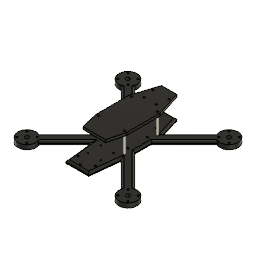
Drone Frame (Autodesk Fusion 360 design; units mm, degrees)
Autodesk Fusion 360 part; units mm, degrees
note: some values were not read from the file. Chosen so that the rebuilt part matches the saved one: which bodies a step acts on; which face or edge a step refers to; which pieces of a blend or face edit are solid. Set by a fixed rule: which sketch regions a step uses.
sketch "Sketch1" plane through (0, 0, 0) normal (0, 0, 1) x (1, 0, 0)
  line L0 (-15.25, 15.25) -> (15.25, 15.25)
  line L1 (15.25, 15.25) -> (15.25, -15.25)
  line L2 (15.25, -15.25) -> (-15.25, -15.25)
  line L3 (-15.25, -15.25) -> (-15.25, 15.25)
  circle A0 centre (-15.25, 15.25) radius 1.5
  circle A1 centre (15.25, 15.25) radius 1.5
  circle A2 centre (-15.25, -15.25) radius 1.5
  circle A3 centre (15.25, -15.25) radius 1.5
  line L4 (-23, 22) -> (0, 22)
  line L5 (-23, 22) -> (23, 22)
  line L6 (23, 22) -> (23, -22)
  line L7 (23, -22) -> (-23, -22)
  line L8 (-23, -22) -> (-23, 22)
  line L9 (-10, -38) -> (-10, -33)
  line L10 (-10, -33) -> (0, -33)
  line L11 (-10, -33) -> (10, -33)
  line L12 (10, -33) -> (10, -53)
  line L13 (10, -53) -> (-10, -53)
  line L14 (-10, -53) -> (-10, -33)
  circle A4 centre (-10, -33) radius 1
  circle A5 centre (10, -33) radius 1
  circle A6 centre (-10, -53) radius 1
  circle A7 centre (10, -53) radius 1
  line L15 (9.6, 35) -> (-9.6, 35)
  circle A8 centre (-9.6, 35) radius 1.5
  circle A9 centre (9.6, 35) radius 1.5
  circle A10 centre (0, 0) radius 112.5
  line L16 (0, 0) -> (-79.5495, -79.5495)
  line L17 (0, 0) -> (-79.5495, 79.5495)
  line L18 (0, 0) -> (79.5495, 79.5495)
  line L19 (0, 0) -> (79.5495, -79.5495)
  line L20 (0, 112.5) -> (0, -112.5)
  line L21 (-87.5495, -71.5495) -> (-71.5495, -71.5495)
  line L22 (-71.5495, -71.5495) -> (-71.5495, -87.5495)
  line L23 (-71.5495, -87.5495) -> (-87.5495, -87.5495)
  line L24 (-87.5495, -87.5495) -> (-87.5495, -71.5495)
  line L25 (-87.5495, -71.5495) -> (-71.5495, -87.5495) construction
  line L26 (-71.5495, -71.5495) -> (-87.5495, -87.5495) construction
  line L27 (-87.5495, 87.5495) -> (-71.5495, 87.5495)
  line L28 (-71.5495, 87.5495) -> (-71.5495, 71.5495)
  line L29 (-71.5495, 71.5495) -> (-87.5495, 71.5495)
  line L30 (-87.5495, 71.5495) -> (-87.5495, 87.5495)
  line L31 (-87.5495, 87.5495) -> (-71.5495, 71.5495) construction
  line L32 (-71.5495, 87.5495) -> (-87.5495, 71.5495) construction
  line L33 (71.5495, 87.5495) -> (87.5495, 87.5495)
  line L34 (87.5495, 87.5495) -> (87.5495, 71.5495)
  line L35 (87.5495, 71.5495) -> (71.5495, 71.5495)
  line L36 (71.5495, 71.5495) -> (71.5495, 87.5495)
  line L37 (71.5495, 87.5495) -> (87.5495, 71.5495) construction
  line L38 (87.5495, 87.5495) -> (71.5495, 71.5495) construction
  line L39 (71.5495, -71.5495) -> (87.5495, -71.5495)
  line L40 (87.5495, -71.5495) -> (87.5495, -87.5495)
  line L41 (87.5495, -87.5495) -> (71.5495, -87.5495)
  line L42 (71.5495, -87.5495) -> (71.5495, -71.5495)
  line L43 (71.5495, -71.5495) -> (87.5495, -87.5495) construction
  line L44 (87.5495, -71.5495) -> (71.5495, -87.5495) construction
  circle A11 centre (-87.5495, 87.5495) radius 1.5
  circle A12 centre (-71.5495, 87.5495) radius 1.5
  circle A13 centre (-87.5495, 71.5495) radius 1.5
  circle A14 centre (-71.5495, 71.5495) radius 1.5
  circle A15 centre (71.5495, 87.5495) radius 1.5
  circle A16 centre (87.5495, 87.5495) radius 1.5
  circle A17 centre (71.5495, 71.5495) radius 1.5
  circle A18 centre (87.5495, 71.5495) radius 1.5
  circle A19 centre (-87.5495, -71.5495) radius 1.5
  circle A20 centre (-71.5495, -71.5495) radius 1.5
  circle A21 centre (-87.5495, -87.5495) radius 1.5
  circle A22 centre (-71.5495, -87.5495) radius 1.5
  circle A23 centre (71.5495, -71.5495) radius 1.5
  circle A24 centre (87.5495, -71.5495) radius 1.5
  circle A25 centre (71.5495, -87.5495) radius 1.5
  circle A26 centre (87.5495, -87.5495) radius 1.5
  circle A27 centre (-79.5495, -79.5495) radius 3
  circle A28 centre (-79.5495, 79.5495) radius 3
  circle A29 centre (79.5495, 79.5495) radius 3
  circle A30 centre (79.5495, -79.5495) radius 3
  circle A31 centre (-79.5495, 79.5495) radius 14.5
  circle A32 centre (79.5495, 79.5495) radius 14.5
  circle A33 centre (-79.5495, -79.5495) radius 14.5
  circle A34 centre (79.5495, -79.5495) radius 14.5
  line L45 (24, 25) -> (-24, 25)
  line L46 (-24, 25) -> (-24, -25)
  line L47 (-24, -25) -> (24, -25)
  line L48 (24, -25) -> (24, 25)
  line L49 (24, 25) -> (-24, -25) construction
  line L50 (-24, 25) -> (24, -25) construction
  line L51 (18, -80) -> (-18, -80)
  line L52 (-24, -25) -> (-18, -80)
  line L53 (24, -25) -> (18, -80)
  line L54 (12, 65) -> (-12, 65)
  line L55 (-12, 65) -> (-24, 25)
  line L56 (12, 65) -> (24, 25)
  line L57 (-76.0778, 65.4712) -> (-24, 13.3934)
  line L58 (-65.4712, 76.0778) -> (-24, 34.6066)
  line L59 (-24, 34.6066) -> (-21.7831, 32.3897)
  line L60 (65.4712, 76.0778) -> (24, 34.6066)
  line L61 (76.0778, 65.4712) -> (24, 13.3934)
  line L62 (24, 34.6066) -> (21.7831, 32.3897)
  line L63 (-76.0778, -65.4712) -> (-24, -13.3934)
  line L64 (-65.4712, -76.0778) -> (-24, -34.6066)
  line L65 (-24, -34.6066) -> (-23.0551, -33.6617)
  line L66 (65.4712, -76.0778) -> (24, -34.6066)
  line L67 (76.0778, -65.4712) -> (24, -13.3934)
  line L68 (24, -34.6066) -> (23.0551, -33.6617)
  circle A35 centre (-20.5, -26) radius 1.5
  line L69 (-16.75, -26.25) -> (16.75, -26.25)
  line L70 (16.75, -26.25) -> (16.75, -59.75)
  line L71 (16.75, -59.75) -> (-16.75, -59.75)
  line L72 (-16.75, -59.75) -> (-16.75, -26.25)
  line L73 (-16.75, -26.25) -> (16.75, -59.75) construction
  line L74 (16.75, -26.25) -> (-16.75, -59.75) construction
  circle A36 centre (20.5, -26) radius 1.5
  circle A37 centre (-20.5, 26) radius 1.5
  circle A38 centre (20.5, 26) radius 1.5
  circle A39 centre (-79.5495, -79.5495) radius 63.5
  circle A40 centre (-79.5495, 79.5495) radius 63.5
  circle A41 centre (79.5495, 79.5495) radius 63.5
  circle A42 centre (79.5495, -79.5495) radius 63.5
  circle A43 centre (-13.5, -65) radius 1.5
  circle A44 centre (13.5, -65) radius 1.5
  circle A45 centre (-79.5495, 79.5495) radius 62.5
  circle A46 centre (79.5495, 79.5495) radius 62.5
  circle A47 centre (-79.5495, -79.5495) radius 62.5
  circle A48 centre (79.5495, -79.5495) radius 62.5
  circle A49 centre (0, -75) radius 1.5
  point P0 (0, -43)
  point P1 (0, -43)
  point P2 (0, -43)
  point P3 (0, 35)
  point P4 (-79.5495, -79.5495)
  point P5 (-79.5495, 79.5495)
  point P6 (79.5495, 79.5495)
  point P7 (79.5495, -79.5495)
  point P8 (0, -80)
  point P9 (0, 65)
  point P10 (-20.5, -26)
  point P11 (0, -43)
  point P12 (20.5, -26)
  point P13 (-20.5, 26)
  point P14 (20.5, 26)
  point P15 (13.5, -65)
  point P16 (-13.5, -65)
  dimension "d1" = 30.5
  dimension "d2" = 30.5
  dimension "d3" = 15.25
  dimension "d4" = 15.25
  dimension "d5" = 3
  dimension "d6" = 3
  dimension "d7" = 3
  dimension "d8" = 3
  dimension "d18" = 44
  dimension "d19" = 46
  dimension "d20" = 43
  dimension "d24" = 20
  dimension "d25" = 20
  dimension "d26" = 2
  dimension "d27" = 2
  dimension "d28" = 2
  dimension "d29" = 2
  dimension "d30" = 19.2
  dimension "d31" = 35
  dimension "d32" = 3
  dimension "d33" = 3
  dimension "d34" = 225
  dimension "d35" = 90
  dimension "d36" = 90
  dimension "d37" = 90
  dimension "d38" = 45
  dimension "d42" = 16
  dimension "d43" = 16
  dimension "d44" = 16
  dimension "d45" = 16
  dimension "d46" = 16
  dimension "d47" = 16
  dimension "d48" = 16
  dimension "d49" = 16
  dimension "d50" = 3
  dimension "d51" = 3
  dimension "d52" = 3
  dimension "d53" = 3
  dimension "d54" = 3
  dimension "d55" = 3
  dimension "d56" = 3
  dimension "d57" = 3
  dimension "d58" = 3
  dimension "d59" = 3
  dimension "d60" = 3
  dimension "d61" = 3
  dimension "d62" = 3
  dimension "d63" = 3
  dimension "d64" = 3
  dimension "d65" = 3
  dimension "d66" = 6
  dimension "d67" = 6
  dimension "d68" = 6
  dimension "d69" = 6
  dimension "d70" = 29
  dimension "d71" = 29
  dimension "d72" = 29
  dimension "d73" = 29
  dimension "d75" = 50
  dimension "d76" = 48
  dimension "d77" = 36
  dimension "d78" = 55
  dimension "d79" = 24
  dimension "d80" = 40
  dimension "d82" = 15
  dimension "d84" = 15
  dimension "d85" = 15
  dimension "d86" = 15
  dimension "d91" = 23
  dimension "d92" = 20.5
  dimension "d93" = 26
  dimension "d94" = 3
  dimension "d95" = 33.5
  dimension "d96" = 33.5
  dimension "d97" = 6.75
  dimension "d98" = 20.5
  dimension "d99" = 26
  dimension "d100" = 3
  dimension "d101" = 26
  dimension "d102" = 20.5
  dimension "d103" = 26
  dimension "d104" = 20.5
  dimension "d105" = 3
  dimension "d106" = 3
  dimension "d107" = 13.5
  dimension "d108" = 65
  dimension "d109" = 127
  dimension "d110" = 127
  dimension "d111" = 127
  dimension "d112" = 127
  dimension "d113" = 65
  dimension "d114" = 13.5
  dimension "d115" = 3
  dimension "d116" = 3
  dimension "d127" = 125
  dimension "d128" = 125
  dimension "d129" = 125
  dimension "d130" = 125
  dimension "d142" = 3
  dimension "d143" = 10
  dimension "d144" = 10
  dimension "d145" = 13.5
  dimension "d146" = 13.5
  constraint horizontal L0
  constraint vertical L1
  constraint horizontal L2
  constraint vertical L3
  constraint coincident L0.start L3.end
  constraint coincident L0.end L1.start
  constraint coincident L2.end L3.start
  constraint coincident L1.end L2.start
  constraint horizontal L5
  constraint vertical L6
  constraint horizontal L7
  constraint vertical L8
  constraint coincident P11 P2
  constraint horizontal L11
  constraint vertical L12
  constraint horizontal L13
  constraint vertical L14
  constraint coincident L9.end L10.start
  constraint coincident L11.end L12.start
  constraint coincident L13.end L14.start
  constraint coincident L12.end L13.start
  constraint midpoint L15 P3
  constraint parallel L5 L15
  constraint coincident L15.end A8.centre
  constraint coincident L15.start A9.centre
  constraint coincident A10.centre L16.start
  constraint coincident A10 P4
  constraint coincident A10 P5
  constraint coincident A10 P6
  constraint coincident A10 P7
  constraint coincident A10 L20.start
  constraint coincident A10 L20.end
  constraint perpendicular L4 L20
  constraint horizontal L21
  constraint perpendicular L21 L22
  constraint parallel L21 L23
  constraint parallel L22 L24
  constraint coincident L25 P4
  constraint coincident L26 P4
  constraint coincident P4 L16.end
  constraint horizontal L27
  constraint perpendicular L27 L28
  constraint parallel L27 L29
  constraint parallel L28 L30
  constraint coincident L31 P5
  constraint coincident L32 P5
  constraint coincident P5 L17.end
  constraint horizontal L33
  constraint perpendicular L33 L34
  constraint parallel L33 L35
  constraint parallel L34 L36
  constraint coincident L37 P6
  constraint coincident L38 P6
  constraint coincident P6 L18.end
  constraint horizontal L39
  constraint perpendicular L39 L40
  constraint parallel L39 L41
  constraint parallel L40 L42
  constraint coincident L43 P7
  constraint coincident L44 P7
  constraint coincident P7 L19.end
  constraint coincident L27.start L30.end
  constraint coincident L27.end L28.start
  constraint coincident L29.end L30.start
  constraint coincident L28.end L29.start
  constraint coincident L33.start L36.end
  constraint coincident L33.end L34.start
  constraint coincident L35.end L36.start
  constraint coincident L34.end L35.start
  constraint coincident L21.start L24.end
  constraint coincident L21.end L22.start
  constraint coincident L23.end L24.start
  constraint coincident L22.end L23.start
  constraint coincident L39.start L42.end
  constraint coincident L39.end L40.start
  constraint coincident L41.end L42.start
  constraint coincident L40.end L41.start
  constraint concentric A27 A33
  constraint horizontal L45
  constraint perpendicular L45 L46
  constraint parallel L45 L47
  constraint parallel L46 L48
  constraint coincident L49 A10.centre
  constraint coincident L50 A10.centre
  constraint midpoint L51 P8
  constraint coincident L20 P8
  constraint perpendicular L20 L51
  constraint coincident A10.centre L20
  constraint midpoint L54 P9
  constraint coincident L20 P9
  constraint perpendicular L20 L54
  constraint coincident A31 L57.start
  constraint coincident L46 L57.end
  constraint coincident A31 L58.start
  constraint coincident L46 L58.end
  constraint parallel L57 L58
  constraint coincident L55 L59.end
  constraint parallel L58 L59
  constraint coincident A32 L60.start
  constraint coincident L48 L60.end
  constraint coincident A32 L61.start
  constraint coincident L48 L61.end
  constraint parallel L60 L61
  constraint coincident L56 L62.end
  constraint parallel L60 L62
  constraint coincident A33 L63.start
  constraint coincident L46 L63.end
  constraint coincident A33 L64.start
  constraint coincident L46 L64.end
  constraint parallel L63 L64
  constraint coincident L52 L65.end
  constraint parallel L64 L65
  constraint coincident A34 L66.start
  constraint coincident L48 L66.end
  constraint coincident A34 L67.start
  constraint coincident L48 L67.end
  constraint parallel L66 L67
  constraint coincident L53 L68.end
  constraint parallel L66 L68
  constraint coincident P10 A35.centre
  constraint horizontal L69
  constraint perpendicular L69 L70
  constraint parallel L69 L71
  constraint parallel L70 L72
  constraint coincident L73 P11
  constraint coincident L74 P11
  constraint coincident P11 L20
  constraint coincident P12 A36.centre
  constraint coincident P13 A37.centre
  constraint coincident P14 A38.centre
  constraint concentric A27 A39
  constraint concentric A29 A41
  constraint coincident P16 A43.centre
  constraint coincident P15 A44.centre
  constraint concentric A31 A45
  constraint concentric A29 A46
  constraint concentric A27 A47
  constraint concentric A30 A48
  constraint coincident L20 A49.centre
  measures "d1" distance of L0.start L0.end
  measures "d2" distance of L0.start L2.end
  measures "d3" distance of A10.centre L1
  measures "d4" distance of A10.centre L0
  measures "d5" diameter of A0
  measures "d6" diameter of A1
  measures "d7" diameter of A2
  measures "d8" diameter of A3
  measures "d18" distance of L4.start L7.end
  measures "d19" distance of L6.end L7.end
  measures "d20" distance of A10.centre P11
  measures "d24" distance of L9.end L13.end
  measures "d25" distance of L9.end L11.end
  measures "d26" diameter of A4
  measures "d27" diameter of A5
  measures "d28" diameter of A6
  measures "d29" diameter of A7
  measures "d30" distance of L15.start L15.end
  measures "d31" distance of A10.centre P3
  measures "d32" diameter of A8
  measures "d33" diameter of A9
  measures "d34" diameter of A10
  measures "d35" angle of L16 L17
  measures "d36" angle of L17 L18
  measures "d37" angle of L18 L19
  measures "d38" angle of L17 L20
  measures "d42" distance of L21.end L22.end
  measures "d43" distance of L22.end L23.end
  measures "d44" distance of L27.end L28.end
  measures "d45" distance of L27.start L27.end
  measures "d46" distance of L33.end L34.end
  measures "d47" distance of L33.start L33.end
  measures "d48" distance of L39.end L40.end
  measures "d49" distance of L40.end L41.end
  measures "d50" diameter of A11
  measures "d51" diameter of A12
  measures "d52" diameter of A13
  measures "d53" diameter of A14
  measures "d54" diameter of A15
  measures "d55" diameter of A16
  measures "d56" diameter of A17
  measures "d57" diameter of A18
  measures "d58" diameter of A19
  measures "d59" diameter of A20
  measures "d60" diameter of A21
  measures "d61" diameter of A22
  measures "d62" diameter of A23
  measures "d63" diameter of A24
  measures "d64" diameter of A25
  measures "d65" diameter of A26
  measures "d66" diameter of A27
  measures "d67" diameter of A28
  measures "d68" diameter of A29
  measures "d69" diameter of A30
  measures "d70" diameter of A31
  measures "d71" diameter of A32
  measures "d72" diameter of A33
  measures "d73" diameter of A34
  measures "d75" distance of L45.end L46.end
  measures "d76" distance of L45.start L45.end
  measures "d77" distance of L51.start L51.end
  measures "d78" distance of L47 L51
  measures "d79" distance of L54.start L54.end
  measures "d80" distance of L45 L54
  measures "d82" distance of L57 L58
  measures "d84" distance of L60 L61
  measures "d85" distance of L63 L64
  measures "d86" distance of L66 L67
  measures "d91" distance of A10.centre L8
  measures "d92" horizontal distance of A10.centre P10
  measures "d93" vertical distance of A10.centre P10
  measures "d94" diameter of A35
  measures "d95" distance of L69.end L70.end
  measures "d96" distance of L70.end L71.end
  measures "d97" distance of L13 L71
  measures "d98" horizontal distance of A10.centre P12
  measures "d99" vertical distance of A10.centre P12
  measures "d100" diameter of A36
  measures "d101" vertical distance of A10.centre P13
  measures "d102" horizontal distance of A10.centre P13
  measures "d103" vertical distance of A10.centre P14
  measures "d104" horizontal distance of A10.centre P14
  measures "d105" diameter of A37
  measures "d106" diameter of A38
  measures "d107" horizontal distance of A10.centre P15
  measures "d108" vertical distance of A10.centre P15
  measures "d109" diameter of A39
  measures "d110" diameter of A40
  measures "d111" diameter of A41
  measures "d112" diameter of A42
  measures "d113" vertical distance of A10.centre P16
  measures "d114" horizontal distance of A10.centre P16
  measures "d115" diameter of A43
  measures "d116" diameter of A44
  measures "d127" diameter of A45
  measures "d128" diameter of A46
  measures "d129" diameter of A47
  measures "d130" diameter of A48
  measures "d142" diameter of A49
  measures "d143" vertical distance of P16 A49.centre
  measures "d144" vertical distance of P15 A49.centre
  measures "d145" horizontal distance of P16 A49.centre
  measures "d146" horizontal distance of P15 A49.centre
extrude "Extrude1" add sketch "Sketch1" along normal blind 7 contours L0 A0 L4 L5 L17 L20 | L0 A0 L17 L20 | L3 A0 A2 L16 L17 | L3 A0 A2 L4 L5 L7 L8 L16 L17 | L0 A1 L5 L18 L20 | L0 A1 L18 L20 | L2 A2 L16 L20 | L1 A1 A3 L18 L19 | L2 A3 L19 L20 | L4 L5 L17 L20 L45 L46 A37 | L4 L5 L7 L8 L16 L17 L46 | L5 L18 L20 L45 L48 A38 | L2 A2 L7 L16 L20 | L2 A3 L7 L19 L20 | L17 L46 L57 A40 | L17 L46 L55 L58 L59 A40 | L1 A1 A3 L5 L6 L7 L18 L19 | L5 L6 L7 L18 L19 L48 | L20 L45 L54 L55 A37 | L20 L45 L54 L56 A38 | L7 L16 L20 L46 L47 A35 | L7 L19 L20 L47 L48 A36 | L17 L57 A40 A45 | L17 L58 A40 A45 | L18 L48 L56 L60 L62 A41 | L18 L48 L61 A41 | L45 A38 | L45 A38 | L45 A37 | L45 A37 | L16 L46 L52 L64 L65 A39 | L16 L46 L63 A39 | L20 L47 L51 L53 L69 L70 L71 A36 A42 A49 | L20 L47 L51 L52 A35 L69 L71 L72 A39 A49 | L17 A31 L57 A45 | L17 A31 L58 A45 | L18 L60 A41 A46 | L18 L61 A41 A46 | L16 L64 A39 A47 | L16 L63 A39 A47 | L19 L48 L67 A42 | L19 L48 L53 L66 L68 A42 | L11 L12 L13 A5 A7 L20 L69 L70 L71 | L9 L10 L11 L13 L14 A4 A6 L20 L69 L71 L72 | L47 A35 | L47 A35 | L47 A36 | L47 A36 | A10 L17 L29 A13 A14 A31 | A10 L17 L28 A12 A14 A31 | L18 A32 L60 A46 | L18 A32 L61 A46 | L16 A33 L64 A47 | L16 A33 L63 A47 | L19 L67 A42 A48 | L19 L66 A42 A48 | L9 L10 L11 L13 L14 A4 A6 L20 | L11 L12 L13 A5 A7 L20 | A10 L18 L36 A15 A17 A32 | A10 L18 L35 A17 A18 A32 | A10 L16 L22 A20 A22 A33 | A10 L16 L21 A19 A20 A33 | L51 L52 A39 A47 | L19 A34 L67 A48 | L19 A34 L66 A48 | A10 L17 L29 A13 A14 A28 | A10 L27 L30 A11 A12 A13 A31 | L51 L52 A47 | A10 L19 L39 A23 A24 A34 | A10 L19 L42 A23 A25 A34 | L51 L53 A42 A48 | A10 L17 L28 A12 A14 A28 | A10 L23 L24 A19 A21 A22 A33 | A10 L18 L36 A15 A17 A29 | A10 L18 L35 A17 A18 A29 | A10 L33 L34 A15 A16 A18 A32 | A10 L16 L21 A19 A20 A27 | L51 L53 A48 | A10 L27 L30 A11 A12 A13 A28 | A10 L40 L41 A24 A25 A26 A34 | A10 L16 L22 A20 A22 A27 | A10 L19 L39 A23 A24 A30 | A10 L19 L42 A23 A25 A30 | A10 L23 L24 A19 A21 A22 A27 | A10 L33 L34 A15 A16 A18 A29 | A10 L40 L41 A24 A25 A26 A30 makes body 1
fillet "Fillet1" radius 3 91 edges at (-24, 0, 0) (-24, 0, 7) (-32.1329, -21.5263, 0) (-32.1329, -21.5263, 7) (-40.6219, -30.0153, 0) (-40.6219, -30.0153, 7) (-58.5279, -47.9213, 0) (-58.5279, -47.9213, 7) (-47.9213, -58.5279, 0) (-47.9213, -58.5279, 7) (-30.0153, -40.6219, 0) (-30.0153, -40.6219, 7) (-26.8296, -37.4362, 0) (-26.8296, -37.4362, 7) (-23.5275, -34.1341, 0) (-23.5275, -34.1341, 7) (-21.8442, -44.7615, 0) (-21.8442, -44.7615, 7) (-20.4066, -57.9394, 0) (-20.4066, -57.9394, 7) (-19.09, -70.0087, 0) (-19.09, -70.0087, 7) (-17.5256, -80, 0) (-17.5256, -80, 7) (-16.5511, -80, 0) (-16.5511, -80, 7) (-8.0256, -80, 0) (-8.0256, -80, 7) (8.0256, -80, 0) (8.0256, -80, 7) (16.5511, -80, 0) (16.5511, -80, 7) (17.5256, -80, 0) (17.5256, -80, 7) (19.09, -70.0087, 0) (19.09, -70.0087, 7) (20.4066, -57.9394, 0) (20.4066, -57.9394, 7) (21.8442, -44.7615, 0) (21.8442, -44.7615, 7) (23.5275, -34.1341, 0) (23.5275, -34.1341, 7) (26.8296, -37.4362, 0) (26.8296, -37.4362, 7) (30.0153, -40.6219, 0) (30.0153, -40.6219, 7) (47.9213, -58.5279, 0) (47.9213, -58.5279, 7) (58.5279, -47.9213, 0) (58.5279, -47.9213, 7) (40.6219, -30.0153, 0) (40.6219, -30.0153, 7) (32.1329, -21.5263, 0) (32.1329, -21.5263, 7) (24, 0, 0) (24, 0, 7) (32.1329, 21.5263, 0) (32.1329, 21.5263, 7) (40.6219, 30.0153, 0) (40.6219, 30.0153, 7) (58.5279, 47.9213, 0) (58.5279, 47.9213, 7) (47.9213, 58.5279, 0) (47.9213, 58.5279, 7) (30.0153, 40.6219, 0) (30.0153, 40.6219, 7) (26.8296, 37.4362, 0) (26.8296, 37.4362, 7) (22.8915, 33.4981, 0) (22.8915, 33.4981, 7) (16.8915, 48.6948, 0) (16.8915, 48.6948, 7) (6, 65, 0) (6, 65, 7) (-6, 65, 0) (-6, 65, 7) (-16.8915, 48.6948, 7) (-22.8915, 33.4981, 0) (-22.8915, 33.4981, 7) (-26.8296, 37.4362, 0) (-26.8296, 37.4362, 7) (-30.0153, 40.6219, 0) (-30.0153, 40.6219, 7) (-47.9213, 58.5279, 0) (-47.9213, 58.5279, 7) (-58.5279, 47.9213, 0) (-58.5279, 47.9213, 7) (-40.6219, 30.0153, 0) (-40.6219, 30.0153, 7) (-32.1329, 21.5263, 0) (-32.1329, 21.5263, 7) on bodies 1
extrude "Extrude2" add sketch "Sketch1" along normal blind 34.5 separate body contours L45 A38 | L45 A38 | L45 A37 | L45 A37 | L47 A35 | L47 A35 | L47 A36 | L47 A36 makes body 2 at (19.0019, -25.9252, 23) makes body 3 at (21.9925, 26.1494, 23) makes body 4 at (-19.0075, -25.8506, 23) makes body 5 at (-19.0075, 26.1494, 23)
sketch "Sketch2" plane through (0, 0, 7) normal (0, 0, 1) x (-1, 0, 0)
  circle A0 centre (10, 53) radius 1
  circle A1 centre (-79.5495, -79.5495) radius 3
  circle A2 centre (-10, 53) radius 1
  circle A3 centre (-87.5495, 71.5495) radius 1.5
  circle A4 centre (87.5495, 87.5495) radius 1.5
  circle A5 centre (-79.5495, 79.5495) radius 3
  circle A6 centre (-15.25, -15.25) radius 1.5
  circle A7 centre (-13.5, 65) radius 1.5
  circle A8 centre (87.5495, -71.5495) radius 1.5
  circle A9 centre (87.5495, -87.5495) radius 1.5
  circle A10 centre (71.5495, -71.5495) radius 1.5
  circle A11 centre (15.25, -15.25) radius 1.5
  circle A12 centre (-87.5495, -71.5495) radius 1.5
  circle A13 centre (71.5495, 71.5495) radius 1.5
  circle A14 centre (79.5495, 79.5495) radius 3
  circle A15 centre (-71.5495, -71.5495) radius 1.5
  circle A16 centre (-9.6, -35) radius 1.5
  circle A17 centre (-71.5495, -87.5495) radius 1.5
  circle A18 centre (9.6, -35) radius 1.5
  circle A19 centre (-15.25, 15.25) radius 1.5
  circle A20 centre (15.25, 15.25) radius 1.5
  circle A21 centre (79.5495, -79.5495) radius 3
  circle A22 centre (71.5495, -87.5495) radius 1.5
  circle A23 centre (13.5, 65) radius 1.5
  circle A24 centre (-71.5495, 71.5495) radius 1.5
  circle A25 centre (71.5495, 87.5495) radius 1.5
  circle A26 centre (-71.5495, 87.5495) radius 1.5
  circle A27 centre (87.5495, 71.5495) radius 1.5
  circle A28 centre (-87.5495, 87.5495) radius 1.5
  circle A29 centre (-10, 33) radius 1
  circle A30 centre (-87.5495, -87.5495) radius 1.5
  circle A31 centre (10, 33) radius 1
  line L0 (20.3529, -26.7168) -> (66.6207, -72.9847)
  arc A32 (66.6207, -72.9847) -> (72.9847, -66.6207) centre (79.5495, -79.5495) ccw
  line L1 (72.9847, -66.6207) -> (21, -14.636)
  line L2 (21, -14.636) -> (21, 14.636)
  line L3 (21, 14.636) -> (72.9847, 66.6207)
  arc A33 (72.9847, 66.6207) -> (66.6207, 72.9847) centre (79.5495, 79.5495) ccw
  line L4 (66.6207, 72.9847) -> (20.7514, 27.1154)
  line L5 (15.3095, 77) -> (-15.3095, 77)
  line L6 (-15.3095, 77) -> (-20.7514, 27.1154)
  line L7 (-20.7514, 27.1154) -> (-66.6207, 72.9847)
  arc A34 (-66.6207, 72.9847) -> (-72.9847, 66.6207) centre (-79.5495, 79.5495) ccw
  line L8 (-72.9847, 66.6207) -> (-21, 14.636)
  line L9 (-21, 14.636) -> (-21, -14.636)
  line L10 (-21, -14.636) -> (-72.9847, -66.6207)
  arc A35 (-72.9847, -66.6207) -> (-66.6207, -72.9847) centre (-79.5495, -79.5495) ccw
  line L11 (-66.6207, -72.9847) -> (-20.3529, -26.7168)
  line L12 (-20.3529, -26.7168) -> (-9.7679, -62)
  line L13 (-9.7679, -62) -> (9.7679, -62)
  line L14 (9.7679, -62) -> (20.3529, -26.7168)
  circle A36 centre (-20.5, 26) radius 1.5
  circle A37 centre (20.5, 26) radius 1.5
  circle A38 centre (-20.5, -26) radius 1.5
  circle A39 centre (20.5, -26) radius 1.5
  circle A40 centre (9.6, -35) radius 1.5
  circle A41 centre (-9.6, -35) radius 1.5
  line L15 (-12.0604, -64.9096) -> (11.9396, -64.9096)
  line L16 (11.9396, -64.9096) -> (24.5, -26)
  line L17 (-12.0604, -64.9096) -> (-24.5, -26)
  line L18 (-0.0604, -64.9096) -> (-0.0604, -26)
  line L19 (24.5, -26) -> (24.5, 26)
  line L20 (-24.5, -26) -> (-24.5, 26)
  line L21 (24.5, 26) -> (18, 53)
  line L22 (-24.5, 26) -> (-17.9277, 53)
  line L23 (18, 53) -> (-17.9277, 53)
  circle A42 centre (12.6, -52) radius 1.5
  circle A43 centre (-12.6, -52) radius 1.5
  circle A44 centre (0, 75) radius 1.5
  point P0 (-0.0604, -64.9096)
  point P1 (-0.0604, -26)
  dimension "d120" = 24
  dimension "d125" = 4
  dimension "d126" = 4
  dimension "d133" = 3
  dimension "d134" = 3
  dimension "d135" = 17
  dimension "d136" = 3
  dimension "d137" = 17
  dimension "d138" = 3
  constraint midpoint L15 P0
  constraint parallel L13 L15
  constraint coincident P0 L18.start
  constraint coincident P1 L18.end
  constraint vertical L19
  constraint vertical L20
  constraint coincident L6 L22.end
  measures "d120" distance of L15.start L15.end
  measures "d125" distance of A39.centre L16.end
  measures "d126" distance of A38.centre L17.end
  measures "d133" diameter of A42
  measures "d134" diameter of A43
  measures "d135" vertical distance of A18.centre A42.centre
  measures "d136" horizontal distance of A18.centre A42.centre
  measures "d137" vertical distance of A16.centre A43.centre
  measures "d138" horizontal distance of A16.centre A43.centre
extrude "Extrude3" add sketch "Sketch2" along normal blind 4 from surface at 28 separate body contours A0 A2 L0 L1 L2 L3 L6 L7 L8 L9 L10 L11 L12 L13 L14 A36 A38 A39 L16 L17 L19 L20 L21 L22 L23 A42 A43 | A0 L23 | A2 L23 | L6 L7 A36 L22 | L1 L2 L3 L19 | L6 L7 A36 | L6 L7 A36 | L8 L9 L10 L20 | L0 L13 L14 A39 L15 L16 L18 A42 | L0 L14 A39 | L0 L14 A39 | L11 L12 L13 A38 L15 L17 L18 A43 | L14 A42 | L14 A42 | L11 L12 A38 | L11 L12 A38 | L12 A43 | L12 A43 | A6 | A11 | A19 | A20 | A29 | A31 | A37 picked at (10.3296, 52.6611) picked at (-10.2327, 52.407) makes body 6
extrude "Extrude4" add sketch "Sketch1" along normal blind 1 separate body contours L17 L57 A40 A45 | L17 L58 A40 A45 | A10 L57 A40 A45 | A10 L58 A40 A45 | L18 L60 A41 A46 | L18 L61 A41 A46 | L16 L64 A39 A47 | L16 L63 A39 A47 | A10 A40 A45 | A10 L63 A39 A47 | A10 L60 A41 A46 | A10 L61 A41 A46 | L52 L64 A39 A47 | L19 L67 A42 A48 | L19 L66 A42 A48 | A10 A39 A47 | A10 A41 A46 | A10 L67 A42 A48 | L51 L52 A39 A47 | L53 L66 A42 A48 | A10 L51 A39 A47 | A10 A42 A48 | L51 L53 A42 A48 | A10 L51 A42 A48 makes body 7 at (142.734, -73.227, 0.6667) makes body 8 at (-16.3651, 85.8721, 0.6667) makes body 9 at (-81.1326, -16.0692, 0.6667) makes body 10 at (142.734, 85.8721, 0.6667)
extrude "Extrude5" cut sketch "Sketch2" along normal blind 4 from surface at 28 contours L14 A42 | L14 A42 | L12 A43 | L12 A43 bodies 6
sketch "Sketch3" plane through (0, 0, 0) normal (0, 0, -1) x (1, 0, 0)
  arc A0 (66.6207, -72.9847) -> (72.9847, -66.6207) centre (79.5495, -79.5495) ccw
  line L0 (72.9847, -66.6207) -> (21, -14.636)
  line L1 (21, -14.636) -> (21, 14.636)
  line L2 (21, 14.636) -> (72.9847, 66.6207)
  arc A1 (72.9847, 66.6207) -> (66.6207, 72.9847) centre (79.5495, 79.5495) ccw
  line L3 (66.6207, 72.9847) -> (20.7514, 27.1154)
  line L4 (20.7514, 27.1154) -> (15.3095, 77)
  line L5 (15.3095, 77) -> (-15.3095, 77)
  line L6 (-15.3095, 77) -> (-20.7514, 27.1154)
  line L7 (-20.7514, 27.1154) -> (-66.6207, 72.9847)
  arc A2 (-66.6207, 72.9847) -> (-72.9847, 66.6207) centre (-79.5495, 79.5495) ccw
  line L8 (-72.9847, 66.6207) -> (-21, 14.636)
  line L9 (-21, 14.636) -> (-21, -14.636)
  line L10 (-21, -14.636) -> (-72.9847, -66.6207)
  arc A3 (-72.9847, -66.6207) -> (-66.6207, -72.9847) centre (-79.5495, -79.5495) ccw
  line L11 (-22.7622, -29.1261) -> (-12.9, -62)
  line L12 (-12.9, -62) -> (9.7679, -62)
  line L13 (9.7679, -62) -> (20.3529, -26.7168)
  line L14 (20.3529, -26.7168) -> (66.6207, -72.9847)
  circle A4 centre (-87.5495, -87.5495) radius 1.5
  circle A5 centre (-13.5, 65) radius 1.5
  circle A6 centre (-71.5495, -87.5495) radius 1.5
  circle A7 centre (71.5495, -71.5495) radius 1.5
  circle A8 centre (87.5495, -87.5495) radius 1.5
  circle A9 centre (71.5495, 87.5495) radius 1.5
  circle A10 centre (-15.25, -15.25) radius 1.5
  circle A11 centre (87.5495, 71.5495) radius 1.5
  circle A12 centre (0, 75) radius 1.5
  circle A13 centre (-87.5495, 87.5495) radius 1.5
  circle A14 centre (71.5495, -87.5495) radius 1.5
  circle A15 centre (15.25, 15.25) radius 1.5
  circle A16 centre (9.6, -35) radius 1.5
  circle A17 centre (-15.25, 15.25) radius 1.5
  circle A18 centre (-10, 53) radius 1
  circle A19 centre (10, 33) radius 1
  circle A20 centre (-79.5495, 79.5495) radius 3
  circle A21 centre (10, 53) radius 1
  circle A22 centre (-71.5495, 71.5495) radius 1.5
  circle A23 centre (-10, 33) radius 1
  circle A24 centre (-9.6, -35) radius 1.5
  circle A25 centre (15.25, -15.25) radius 1.5
  circle A26 centre (-71.5495, 87.5495) radius 1.5
  circle A27 centre (-87.5495, 71.5495) radius 1.5
  circle A28 centre (71.5495, 71.5495) radius 1.5
  circle A29 centre (87.5495, 87.5495) radius 1.5
  circle A30 centre (79.5495, 79.5495) radius 3
  circle A31 centre (87.5495, -71.5495) radius 1.5
  circle A32 centre (79.5495, -79.5495) radius 3
  circle A33 centre (13.5, 65) radius 1.5
  circle A34 centre (-87.5495, -71.5495) radius 1.5
  circle A35 centre (-79.5495, -79.5495) radius 3
  circle A36 centre (-71.5495, -71.5495) radius 1.5
  circle A37 centre (15.25, -15.25) radius 3.25
  circle A38 centre (-15.25, -15.25) radius 3.25
  circle A39 centre (15.25, 15.25) radius 3.25
  circle A40 centre (-15.25, 15.25) radius 3.25
  line L15 (-66.6207, -72.9847) -> (-22.7622, -29.1261)
  dimension "d147" = 6.5
  dimension "d148" = 6.5
  dimension "d149" = 6.5
  dimension "d150" = 6.5
  constraint concentric A25 A37
  constraint concentric A10 A38
  constraint concentric A15 A39
  constraint concentric A17 A40
  measures "d147" diameter of A37
  measures "d148" diameter of A38
  measures "d149" diameter of A39
  measures "d150" diameter of A40
extrude "Extrude6" cut sketch "Sketch3" against normal blind 3 contours A37 | A38 | A39 | A40 bodies 1
fillet "Fillet2" radius 1 4 edges at (12.2199, -16.4253, 0) (12.2199, 14.0747, 0) (-18.2801, -16.4253, 0) (-18.2801, 14.0747, 0) on bodies 1
extrude "Extrude7" cut sketch "Sketch2" along normal blind 4 from surface at 28 contours L6 L7 A36 | L6 L7 A36 | L0 L14 A39 | L0 L14 A39 | L11 L12 A38 | L11 L12 A38 | A37 bodies 6
extrude "Extrude8" cut sketch "Sketch2" against normal blind 25 contours L6 L7 A36 | L6 L7 A36 | L0 L14 A39 | L0 L14 A39 | L11 L12 A38 | L11 L12 A38 | A37 bodies 1
hidden bodies 7 8 9 10
